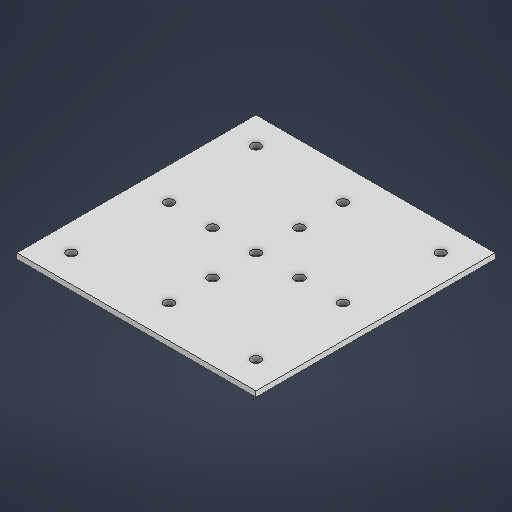
# Autodesk Inventor part: DIFF_HOUSING_TOP
Saved by Autodesk Inventor 2026.1 (Build 301233020, 233B)
## iProperties
Created: 2023-11-30
Part Number: DIFF_HOUSING_TOP
Material: Generic
Document SubType Name: Modeling
Designer: bugme
Density: 1 g/cm^3
Appearance: Default
Author: bugme
Autodesk Inventor part; units mm, degrees
ref_plane "YZ Plane" through (0, 0, 0) normal (1, 0, 0) x (0, 1, 0)
ref_plane "XZ Plane" through (0, 0, 0) normal (0, 1, 0) x (-1, 0, 0)
ref_plane "XY Plane" through (0, 0, 0) normal (0, 0, 1) x (1, 0, 0)
sketch "Sketch1" plane through (0, 0, 0) normal (0, 1, 0) x (-1, 0, 0)
  line L0 (69.85, 69.85) -> (-69.85, 69.85)
  line L1 (-69.85, 69.85) -> (-69.85, -69.85)
  line L2 (-69.85, -69.85) -> (69.85, -69.85)
  line L3 (69.85, -69.85) -> (69.85, 69.85)
  line L4 (97.79, 0) -> (-97.79, 0) projected
  line L5 (0, -97.79) -> (0, 97.79) projected
  point P0 (0, 0)
  dimension "d0" = 139.7
  dimension "d1" = 139.7
  constraints: 8 end point, 2 parallel, 2 symmetric about line, 1 horizontal, 1 perpendicular
  measures "d0" distance of L2.end L1.end
  measures "d1" distance of L0.end L1.end
extrude "Extrusion1" add sketch "Sketch1" along normal blind 3.175
sketch "Sketch2" plane through (0, 3.175, 0) normal (0, 1, 0) x (1, 0, 0)
  line L0 (-69.85, 69.85) -> (-69.85, -69.85) projected
  line L1 (-69.85, -69.85) -> (-69.85, -53.975)
  line L2 (-69.85, -53.975) -> (-53.975, -53.975)
  point P0 (0, 0)
  dimension "d4" = 15.875
  dimension "d5" = 15.875
  constraints: 4 end point, 1 perpendicular, 1 point on line
  measures "d4" distance of L0.end L1.end
  measures "d5" distance of L1.end L2.end
hole "Hole1" at (-53.975, 3.175, 53.975) direction (0, -1, 0) diameter 5.5118 depth 14.1986 tip angle 118 clearance for "Flat Head Machine Screw" size "M5" standard "Ansi Metric M Profile"
mirror "Mirror4" about plane through (0, 0, 0) normal (0, 0, 1) of "Hole1"
mirror "Mirror5" about plane through (0, 0, 0) normal (1, 0, 0) of "Hole1", "Mirror4"
sketch "Sketch5" plane through (0, 3.175, 0) normal (0, 1, 0) x (1, 0, 0)
  point P0 (0, 0)
  point P1 (0, 0)
  constraints: 1 coincident
hole "Hole3" at (0, 3.175, 0) direction (0, -1, 0) diameter 5.5118 end through all
pattern_linear "Rectangular Pattern2" count 5 spacing 25.4 along (1, 0, 0) of "Hole3" first direction both ways yes
pattern_linear "Rectangular Pattern3" count 5 spacing 25.4 along (0, 0, 1) of "Hole3" first direction both ways yes
equation "\"d0\" = d1"
equation "\"d4\" = d5"
body "Solid1"
